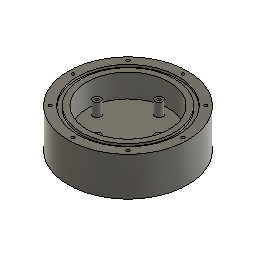
e314 base v4 (Autodesk Fusion 360 design; units mm, degrees)
Autodesk Fusion 360 part; units mm, degrees
sketch "BaseSketch" plane through (0, 0, 0) normal (0, 1, 0) x (1, 0, 0)
  circle A0 centre (0, 0) radius 38.5
  circle A1 centre (0, 0) radius 26.5
  dimension "d1" = 77
  dimension "d2" = 53
  constraint coincident A0.centre A1.centre
  constraint concentric A0 A1
  measures "d1" diameter of A0
  measures "d2" diameter of A1
extrude "Extrude1" add sketch "BaseSketch" against normal blind 10 contours A0 | A1
extrude "Extrude2" add sketch "BaseSketch" along normal blind 15
sketch "ORingSketch" plane through (0, 15, 0) normal (0, 1, 0) x (-1, 0, 0)
  circle A0 centre (0, 0) radius 26.5
  circle A1 centre (0, 0) radius 38.5
  circle A2 centre (0, 0) radius 30
  circle A3 centre (0, 0) radius 32.5
  dimension "d10" = 60
  dimension "d11" = 65
  constraint concentric A0 A2
  constraint concentric A2 A3
  measures "d10" diameter of A2
  measures "d11" diameter of A3
extrude "Extrude3" cut sketch "ORingSketch" against normal blind 1.5 contours A3
sketch "ScrewSketch" plane through (0, 15, 0) normal (0, 1, 0) x (-1, 0, 0)
  circle A0 centre (0, 0) radius 38.5
  circle A1 centre (0, 0) radius 32.5
  circle A2 centre (-35.5, 0) radius 0.95
  circle A3 centre (-25.1023, -25.1023) radius 0.95
  circle A4 centre (0, -35.5) radius 0.95
  circle A5 centre (25.1023, -25.1023) radius 0.95
  circle A6 centre (35.5, 0) radius 0.95
  circle A7 centre (25.1023, 25.1023) radius 0.95
  circle A8 centre (0, 35.5) radius 0.95
  circle A9 centre (-25.1023, 25.1023) radius 0.95
  dimension "d16" = 1.9
  dimension "d19" = 360
  dimension "d22" = 35.5
  constraint horizontal A0.centre A2.centre
  measures "d16" diameter of A2
  measures "d22" distance of A0.centre A2.centre
extrude "Extrude4" cut sketch "ScrewSketch" against normal blind 15 contours A2 | A3 | A4 | A5 | A6 | A7 | A8 | A9
sketch "StandoffSketch" plane through (0, 0, 0) normal (0, 1, 0) x (-1, 0, 0)
  circle A0 centre (0, 0) radius 26.5
  circle A1 centre (0, 0) radius 25
  circle A2 centre (-20, 0) radius 0.95
  circle A3 centre (-20, 0) radius 2.45
  circle A4 centre (0, -20) radius 0.95
  circle A5 centre (0, -20) radius 2.45
  circle A6 centre (20, 0) radius 0.95
  circle A7 centre (20, 0) radius 2.45
  circle A8 centre (0, 20) radius 0.95
  circle A9 centre (0, 20) radius 2.45
  dimension "d25" = 50
  dimension "d27" = 1.9
  dimension "d28" = 20
  dimension "d29" = 4.9
  dimension "d31" = 360
  constraint concentric A0 A1
  constraint horizontal A0.centre A2.centre
  constraint concentric A2 A3
  measures "d25" diameter of A1
  measures "d27" diameter of A2
  measures "d28" distance of A0.centre A2.centre
  measures "d29" diameter of A3
extrude "Extrude5" add sketch "StandoffSketch" along normal blind 8.5 contours A3 | A5 | A7 | A9
extrude "Extrude6" cut sketch "StandoffSketch" against normal blind 7 contours A2 | A4 | A6 | A8
ref_plane "WorkPlane1" through (0, 15, 0) normal (0, 1, 0) x (1, 0, 0)
sketch "RubberPlugSketch" plane through (0, 0, 0) normal (0, 1, 0) x (-1, 0, 0)
  circle A0 centre (20, 0) radius 2.45
  circle A1 centre (0, -20) radius 2.45
  circle A2 centre (0, 0) radius 26.5
  circle A3 centre (-20, 0) radius 2.45
  circle A4 centre (0, 20) radius 2.45
  circle A5 centre (-13.9903, 13.5103) radius 6.25
  line L0 (0, 0) -> (-26.5, 0) construction
  line L1 (0, 0) -> (-13.9903, 13.5103) construction
  dimension "d37" = 12.5
  dimension "d38" = 19.4488
  dimension "d39" = 44
  constraint coincident A2.centre L0.start
  constraint coincident A2 L0.end
  constraint horizontal L0
  constraint coincident A5.centre L1.end
  measures "d37" diameter of A5
  measures "d38" distance of A2.centre A5.centre
  measures "d39" angle of L0 L1
extrude "Extrude7" cut sketch "RubberPlugSketch" against normal blind 10 contours A5
equation "d1 = diameter"
equation "d2 = PCBdiameter + tolerance"
equation "tolerance = 3 mm"
equation "d4 = -CaseBottomThick"
equation "CaseBottomThick = 10 mm"
equation "height = 25 mm"
equation "d8 = height - CaseBottomThick"
equation "d10 = d11 - 5 mm"
equation "diameter = 77 mm"
equation "screwDiameter = 1.9 mm"
equation "d16 = screwDiameter"
equation "screwDepth = 15 mm"
equation "d22 = diameter / 2 - 3 mm"
equation "d23 = -screwDepth"
equation "d25 = PCBdiameter"
equation "PCBdiameter = 50 mm"
equation "d27 = screwDiameter"
equation "d28 = PCBdiameter / 2 - 5 mm"
equation "d29 = screwDiameter + tolerance"
equation "d32 = 5.5 mm + tolerance"
equation "d34 = -CaseBottomThick + tolerance"
equation "d40 = -CaseBottomThick"
